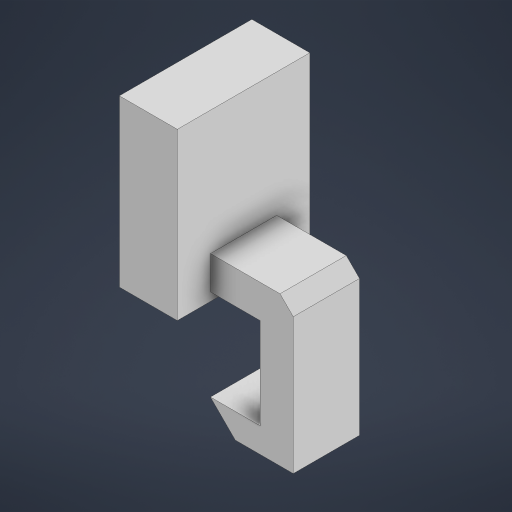
# Autodesk Inventor part: prueba_up
Saved by Autodesk Inventor 2024.1 (Build 281209000, 209)
## iProperties
Created: 2023-07-21
Part Number: prueba_up
Material: Generic
Document SubType Name: Modeling
Designer: LabTel_Admin
Density: 1 g/cm^3
Appearance: Default
Author: LabTel_Admin
Autodesk Inventor part; units mm, degrees
ref_plane "YZ Plane" through (0, 0, 0) normal (1, 0, 0) x (0, 1, 0)
ref_plane "XZ Plane" through (0, 0, 0) normal (0, 1, 0) x (-1, 0, 0)
ref_plane "XY Plane" through (0, 0, 0) normal (0, 0, 1) x (1, 0, 0)
sketch "Sketch1" plane through (0, 0, 0) normal (0, 1, 0) x (-1, 0, 0)
  line L0 (-1.75, -4) -> (1.75, -4)
  line L1 (1.75, -4) -> (1.75, 4)
  line L2 (1.75, 4) -> (-1.75, 4)
  line L3 (-1.75, 4) -> (-1.75, -4)
  line L4 (-1.75, -4) -> (1.75, 4) construction
  line L5 (1.75, -4) -> (-1.75, 4) construction
  point P0 (0, 0)
  dimension "d0" = 3.5
  dimension "d1" = 8
  constraints: 12 end point, 2 midpoint, 2 parallel, 1 horizontal, 1 perpendicular
  measures "d0" distance of L2.end L1.end
  measures "d1" distance of L0.end L1.end
extrude "Extrusion1" add sketch "Sketch1" along normal blind 10
sketch "Sketch2" plane through (1.75, 0, 4) normal (1, 0, 0) x (0, 0, -1)
  line L0 (2, 2.5) -> (6, 2.5)
  line L1 (6, 2.5) -> (6, 0.5)
  line L2 (6, 0.5) -> (2, 0.5)
  line L3 (2, 0.5) -> (2, 2.5)
  line L4 (8, 0) -> (8, 10) projected
  line L5 (0, 0) -> (8, 0) projected
  point P0 (4, 0)
  dimension "d4" = 2
  dimension "d5" = 4
  dimension "d6" = 2
  dimension "d7" = 0.5
  constraints: 8 end point, 2 parallel, 1 horizontal, 1 perpendicular
  measures "d4" distance between parallel lines of L4 L1
  measures "d5" distance of L1.end L2.end
  measures "d6" distance of L2.end L0.start
  measures "d7" distance between parallel lines of L5 L2
extrude "Extrusion2" add sketch "Sketch2" along normal blind 5
sketch "Sketch3" plane through (1.75, 0.5, -2) normal (0, -1, 0) x (1, 0, 0)
  line L0 (5, 4) -> (5, 0) projected
  line L1 (0, 0) -> (5, 0) projected
  line L2 (5, 4) -> (3, 4)
  line L3 (3, 4) -> (3, 0)
  line L4 (3, 0) -> (5, 0)
  line L5 (5, 0) -> (5, 4)
  point P0 (-1.75, 2)
  dimension "d22" = 2
  constraints: 8 end point, 2 parallel, 1 horizontal, 1 perpendicular, 1 point on line
  measures "d22" distance of L4.end L3.end
extrude "Extrusion3" add sketch "Sketch3" along normal blind 7
chamfer "Chamfer1" distance 0.8 angle 45 1 edges at (6.75, 2.5, 0)
sketch "Sketch6" plane through (4.75, 0.5, -2) normal (-1, 0, 0) x (0, 0, 1)
  line L0 (0, -7) -> (4, -7) projected
  line L1 (0, 0) -> (0, -7) projected
  line L2 (4, -7) -> (0, -7)
  line L3 (0, -7) -> (0, -5.5)
  line L4 (0, -5.5) -> (4, -5.5)
  line L5 (4, -5.5) -> (4, -7)
  point P0 (2, -0.5)
  dimension "d23" = 1.5
  constraints: 8 end point, 2 parallel, 1 horizontal, 1 perpendicular, 1 point on line
  measures "d23" distance of L2.end L3.end
extrude "Extrusion6" add sketch "Sketch6" along normal blind 3
chamfer "Chamfer2" distance 1.5 angle 45 1 edges at (1.75, -6.5, 0)
body "Solid1"
